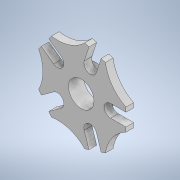
# Autodesk Inventor part: outra cruz de malta
Saved by Autodesk Inventor 2022 (Build 260153000, 153)
## iProperties
Created: 2023-03-13
Part Number: outra cruz de malta
Material: Genérico
Document SubType Name: Modeling
Designer: jpjoa
Density: 1 g/cm^3
Appearance: Padrão
Author: jpjoa
Autodesk Inventor part; units mm, degrees
ref_plane "YZ Plane" through (0, 0, 0) normal (1, 0, 0) x (0, 1, 0)
ref_plane "XZ Plane" through (0, 0, 0) normal (0, 1, 0) x (-1, 0, 0)
ref_plane "XY Plane" through (0, 0, 0) normal (0, 0, 1) x (1, 0, 0)
sketch "Esboço1" plane through (0, 0, 0) normal (0, 0, 1) x (1, 0, 0)
  circle A0 centre (0, 0) radius 15
  circle A1 centre (0, 0) radius 10
  line L0 (18, 0) -> (102.7313, 0) construction
  line L1 (23, -5) -> (97.7313, -5)
  line L2 (97.7313, 5) -> (23, 5)
  arc A2 (23, 5) -> (23, -5) centre (23, 0) ccw
  arc A3 (97.7313, -5) -> (97.7313, 5) centre (97.7313, 0) ccw
  circle A4 centre (-60, 0) radius 30
  line L3 (35, 50) -> (135, 50)
  line L4 (135, 50) -> (135, -50)
  line L5 (135, -50) -> (35, -50)
  line L6 (35, -50) -> (35, 50)
  circle A5 centre (0, 0) radius 75
  circle A6 centre (-18.541, -57.0634) radius 30
  arc A7 (2.3521, 23.4194) -> (11.8627, 20.3292) centre (7.1074, 21.8743) ccw
  line L7 (25.4454, 94.4931) -> (2.3521, 23.4194)
  line L8 (11.8627, 20.3292) -> (34.9559, 91.4029)
  line L9 (58.3684, 17.8361) -> (-36.7372, 48.7378)
  line L10 (-36.7372, 48.7378) -> (-5.8355, 143.8435)
  line L11 (89.2701, 112.9418) -> (58.3684, 17.8361)
  circle A8 centre (48.541, -35.2671) radius 30
  arc A9 (-21.5463, 9.474) -> (-15.6685, 17.5641) centre (-18.6074, 13.5191) ccw
  line L12 (-82.0052, 53.3999) -> (-21.5463, 9.474)
  line L13 (-15.6685, 17.5641) -> (-76.1274, 61.4901)
  line L14 (1.0737, 61.0233) -> (-57.7049, -19.8784)
  line L15 (-57.7049, -19.8784) -> (-138.6066, 38.9002)
  line L16 (-79.828, 119.8019) -> (1.0737, 61.0233)
  circle A10 centre (48.541, 35.2671) radius 30
  arc A11 (-15.6685, -17.5641) -> (-21.5463, -9.474) centre (-18.6074, -13.5191) ccw
  line L17 (-76.1274, -61.4901) -> (-15.6685, -17.5641)
  line L18 (-21.5463, -9.474) -> (-82.0052, -53.3999)
  line L19 (-57.7049, 19.8784) -> (1.0737, -61.0233)
  line L20 (1.0737, -61.0233) -> (-79.828, -119.8019)
  line L21 (-138.6066, -38.9002) -> (-57.7049, 19.8784)
  circle A12 centre (-18.541, 57.0634) radius 30
  arc A13 (11.8627, -20.3292) -> (2.3521, -23.4194) centre (7.1074, -21.8743) ccw
  line L22 (34.9559, -91.4029) -> (11.8627, -20.3292)
  line L23 (2.3521, -23.4194) -> (25.4454, -94.4931)
  line L24 (-36.7372, -48.7378) -> (58.3684, -17.8361)
  line L25 (58.3684, -17.8361) -> (89.2701, -112.9418)
  line L26 (-5.8355, -143.8435) -> (-36.7372, -48.7378)
  point P0 (60.3657, 0)
  point P1 (35, 0)
  point P2 (10.8156, 33.287)
  point P3 (-28.3156, 20.5725)
  point P4 (-28.3156, -20.5725)
  point P5 (10.8156, -33.287)
  point P6 (35, 5)
  point P7 (35, 8.497)
  point P8 (18.8967, 30.6613)
  point P9 (15.5709, 31.7419)
  point P10 (6.0603, 34.8321)
  point P11 (2.7345, 35.9127)
  point P12 (-23.3212, 27.4467)
  point P13 (-25.3767, 24.6176)
  point P14 (-31.2545, 16.5274)
  point P15 (-33.31, 13.6983)
  point P16 (-33.31, -13.6983)
  point P17 (-31.2545, -16.5274)
  point P18 (-25.3767, -24.6176)
  point P19 (-23.3212, -27.4467)
  point P20 (2.7345, -35.9127)
  point P21 (6.0603, -34.8321)
  point P22 (15.5709, -31.7419)
  point P23 (18.8967, -30.6613)
  point P24 (35, -8.497)
  point P25 (35, -5)
  dimension "d0" = 20
  dimension "d1" = 30
  dimension "d2" = 5
  dimension "d3" = 23
  dimension "d4" = 60
  dimension "d5" = 60
  dimension "d6" = 35
  dimension "d7" = 100
  dimension "d8" = 100
  dimension "d9" = 150
  dimension "d10" = 5
  dimension "d11" = 62.7313
  dimension "d14" = 360
  constraints: 56 end point, 14 centre point, 14 point on circle, 4 tangent, 3 horizontal alignment, 3 parallel, 2 coincident, 2 horizontal, 2 midpoint, 2 point on line, 1 concentric, 1 perpendicular, 91 other
  measures "d0" diameter of A1
  measures "d1" diameter of A0
  measures "d2" radius of A2
  measures "d3" distance of A2.centre point (0, 0)
  measures "d4" diameter of A4
  measures "d5" distance of point (0, 0) A4.centre
  measures "d6" distance from line of L6 point (0, 0)
  measures "d7" distance between parallel lines of L5 L3
  measures "d8" distance between parallel lines of L4 L6
  measures "d9" diameter of A5
  measures "d10" radius of A3
  measures "d11" distance of A3.centre point (35, 0)
extrude "Extrusão1" add sketch "Esboço1" along normal blind 6 contours L1 L6 A8 L24 L22 A13 L23 A6 L19 L17 A11 L18 A4 L14 L12 A9 L13 A12 L9 L7 A7 L8 A10 L2 A2
extrude "Extrusão2" add sketch "Esboço1" along normal mid plane 12 contours A0
